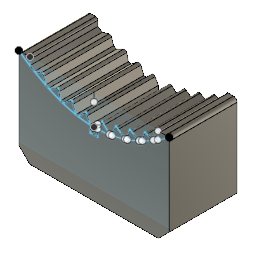
Sliderpot (Autodesk Fusion 360 design; units mm, degrees)
Autodesk Fusion 360 part; units mm, degrees
sketch "Sketch1" plane through (0, 0, 0) normal (0, 0, 1) x (1, 0, 0)
  line L0 (10.5, -4.75) -> (-10.5, -4.75)
  line L1 (-10.5, -4.75) -> (-10.5, 4.75)
  line L2 (-10.5, 4.75) -> (10.5, 4.75)
  line L3 (10.5, 4.75) -> (10.5, -4.75)
  line L4 (10.5, -4.75) -> (-10.5, 4.75) construction
  line L5 (-10.5, -4.75) -> (10.5, 4.75) construction
  dimension "d1" = 21
  dimension "d2" = 9.5
  constraint horizontal L0
  constraint perpendicular L0 L1
  constraint parallel L0 L2
  constraint parallel L1 L3
  constraint coincident L4 origin
  constraint coincident L5 origin
  measures "d1" distance of L1.end L2.end
  measures "d2" distance of L0.end L1.end
extrude "Extrude1" add sketch "Sketch1" along normal blind 11
sketch "Sketch2" plane through (0, 0, 0) normal (0, 0, -1) x (1, 0, 0)
  line L0 (-10.5, -4.75) -> (10.5, -4.75)
  line L1 (10.5, -4.75) -> (10.5, 4.75)
  line L2 (10.5, 4.75) -> (-10.5, 4.75)
  line L3 (-10.5, 4.75) -> (-10.5, -4.75)
  line L4 (2.05, -0.625) -> (-2.05, -0.625)
  line L5 (-2.05, -0.625) -> (-2.05, 0.625)
  line L6 (-2.05, 0.625) -> (2.05, 0.625)
  line L7 (2.05, 0.625) -> (2.05, -0.625)
  line L8 (2.05, -0.625) -> (-2.05, 0.625) construction
  line L9 (-2.05, -0.625) -> (2.05, 0.625) construction
  dimension "d5" = 4.1
  dimension "d6" = 1.25
  constraint horizontal L4
  constraint perpendicular L4 L5
  constraint parallel L4 L6
  constraint parallel L5 L7
  constraint coincident L8 origin
  constraint coincident L9 origin
  measures "d5" distance of L5.end L6.end
  measures "d6" distance of L4.end L5.end
sketch "Sketch3" plane through (0, -4.75, 0) normal (0, -1, 0) x (1, 0, 0)
  line L0 (-10.5, 0) -> (10.5, 0)
  line L1 (10.5, 0) -> (10.5, 11)
  line L2 (10.5, 11) -> (-10.5, 11)
  line L3 (-10.5, 11) -> (-10.5, 0)
  spline S0 degree 5 poles (-10.5, 11) (-10.0801, 10.6955) (-9.2404, 10.113) (-7.9808, 9.3191) (-6.3012, 8.4228) (-4.2016, 7.5911) (-2.1018, 7.0739) (-0.0019, 6.8968) (2.0982, 7.0739) (4.1984, 7.5912) (6.2988, 8.4229) (7.9792, 9.3192) (9.2396, 10.1131) (10.0799, 10.6955) (10.5, 11) knots 0 0 0 0 0 0 0.1 0.2 0.3 0.4 0.5 0.6 0.7 0.8 0.9 1 1 1 1 1 1
  line L4 (-0.0031, 6.9851) -> (-0.0336, 6.9851)
  line L5 (-0.5, 7.0404) -> (-0.5, 6.0404)
  line L6 (-0.5, 6.0404) -> (0.5, 6.0404)
  line L7 (0.5, 6.0404) -> (0.5, 6.9951)
  line L8 (0, 11) -> (0, 10) construction
  line L9 (-0.5, 7.0404) -> (-1.1379, 8.2493)
  line L10 (-1.1379, 8.2493) -> (-2.1854, 7.1728)
  line L11 (-2.5306, 7.2364) -> (-3.0769, 8.6476)
  line L12 (-3.0769, 8.6476) -> (-4.3485, 7.7175)
  line L13 (-4.6784, 7.8304) -> (-4.9948, 9.181)
  line L14 (-4.9948, 9.181) -> (-6.3365, 8.5115)
  line L15 (-6.7604, 8.715) -> (-7.1089, 9.9152)
  line L16 (-7.1089, 9.9152) -> (-8.3208, 9.5633)
  line L17 (-8.9482, 9.9473) -> (-8.9482, 11)
  line L18 (0.5, 6.9951) -> (0.5, 7.565)
  line L19 (0.5, 7.0404) -> (1.1379, 8.2493)
  line L20 (1.1379, 8.2493) -> (2.1854, 7.1728)
  line L21 (2.5306, 7.2364) -> (3.0769, 8.6476)
  line L22 (3.0769, 8.6476) -> (4.3485, 7.7175)
  line L23 (4.6784, 7.8304) -> (4.9948, 9.181)
  line L24 (4.9948, 9.181) -> (6.3365, 8.5115)
  line L25 (6.7604, 8.715) -> (7.1089, 9.9152)
  line L26 (7.1089, 9.9152) -> (8.3208, 9.5633)
  line L27 (8.9482, 9.9473) -> (8.9482, 11)
  point P0 (-0.0031, 6.9851)
  dimension "d10" = 0.5
  dimension "d11" = 1
  dimension "d12" = 1
  constraint coincident L2.end L3.start
  constraint coincident L1.end L2.start
  constraint coincident P0 L4.start
  constraint perpendicular L5 L6
  constraint coincident S0 L7.end
  constraint perpendicular L6 L7
  constraint vertical L5
  constraint midpoint L2 L8.start
  constraint perpendicular L2 L8
  constraint coincident S0 L10.end
  constraint coincident S0 L11.start
  constraint coincident S0 L12.end
  constraint coincident S0 L13.start
  constraint coincident S0 L14.end
  constraint coincident S0 L15.start
  constraint coincident S0 L16.end
  constraint perpendicular L15 L16
  constraint coincident S0 L17.start
  constraint coincident L2 L17.end
  constraint perpendicular L2 L17
  constraint parallel L7 L18
  constraint symmetric L5.start L8 L19.start
  constraint symmetric L8 L9.end L19.end
  constraint symmetric L8 L10.end L20.end
  constraint symmetric L8 L11.start L21.start
  constraint symmetric L8 L11.end L21.end
  constraint symmetric L8 L12.end L22.end
  constraint symmetric L8 L13.start L23.start
  constraint symmetric L8 L13.end L23.end
  constraint symmetric L8 L14.end L24.end
  constraint symmetric L8 L15.start L25.start
  constraint symmetric L8 L15.end L25.end
  constraint symmetric L8 L16.end L26.end
  constraint symmetric L8 L17.start L27.start
  constraint symmetric L8 L17.end L27.end
  measures "d10" distance of P0 L5.start
  measures "d11" distance of L5.start L5.end
  measures "d12" distance of L5.end L6.end
extrude "Extrude2" cut sketch "Sketch2" against normal blind 5 contours L4 L5 L6 L7
extrude "Extrude5" cut sketch "Sketch3" against normal blind 9.5 contours L2 S0 L4 L5 L9 L10 L11 L12 L13 L14 L15 L16 L17 L18 L19 L20 L21 L22 L23 L24 L25 L26 L27 | S0 L4 L5 L6 L7
fillet "Fillet2" radius 0.3 10 edges at (-8.9482, 0, 11) (-7.1089, 0, 9.9152) (-4.9948, 0, 9.181) (-3.0769, 0, 8.6476) (-1.1379, 0, 8.2493) (1.1379, 0, 8.2493) (3.0769, 0, 8.6476) (4.9948, 0, 9.181) (7.1089, 0, 9.9152) (8.9482, 0, 11)
fillet "Fillet3" radius 0.5 2 edges at (10.5, 0, 11) (-10.5, 0, 11)
extrude "Extrude6" add 1 faces at (-7.6833, 0.2083, 0) along direction (0, 0, -1) blind 2
chamfer "Chamfer2" distance 1.5 angle 45 2 edges at (-10.5, 0, -2) (10.5, 0, -2)
